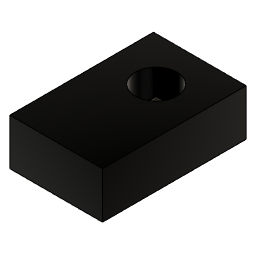
AMS_AS7341 (Autodesk Fusion 360 design; units mm, degrees)
Autodesk Fusion 360 part; units mm, degrees
note: some values were not read from the file. Set by a fixed rule: which face or edge a step refers to.
sketch "Sketch1" plane through (0, 0, 0) normal (0, 0, 1) x (1, 0, 0) in component "Body"
  line L0 (1, -1.55) -> (-1, -1.55)
  line L1 (-1, -1.55) -> (-1, 1.55)
  line L2 (-1, 1.55) -> (1, 1.55)
  line L3 (1, 1.55) -> (1, -1.55)
  line L4 (1, -1.55) -> (-1, 1.55) construction
  line L5 (-1, -1.55) -> (1, 1.55) construction
  dimension "d1" = 2
  dimension "d2" = 3.1
  constraint horizontal L0
  constraint perpendicular L0 L1
  constraint parallel L0 L2
  constraint parallel L1 L3
  constraint coincident L4 origin
  constraint coincident L5 origin
  measures "d1" distance of L1.end L2.end
  measures "d2" distance of L0.end L1.end
extrude "Extrude1" add sketch "Sketch1" along normal blind 1 makes body 1 in component "Body"
sketch "Sketch2" plane through (0, 0, 1) normal (0, 0, 1) x (-1, 0, 0) in component "Body"
  line L0 (-1, -1.55) -> (1, -1.55)
  line L1 (1, -1.55) -> (1, 1.55)
  line L2 (1, 1.55) -> (-1, 1.55)
  line L3 (-1, 1.55) -> (-1, -1.55)
  line L4 (0, 0) -> (0, -1.55) construction
  circle A0 centre (0, -0.609) radius 0.45
  dimension "d5" = 0.9
  dimension "d6" = 0.609
  constraint coincident L4.start origin
  constraint midpoint L0 L4.end
  constraint coincident L4 A0.centre
  measures "d5" diameter of A0
  measures "d6" distance of L4.start A0.centre
extrude "Extrude2" cut sketch "Sketch2" against normal blind 0.6 contours A0 bodies 1 in component "Body"
sketch "Sketch3" plane through (0, 0, 0) normal (0, 0, -1) x (1, 0, 0) in component "Body"
  line L0 (-1, -1.55) -> (1, -1.55)
  line L1 (1, -1.55) -> (1, 1.55)
  line L2 (1, 1.55) -> (-1, 1.55)
  line L3 (-1, 1.55) -> (-1, -1.55)
  line L4 (0, 1.55) -> (0, -1.55) construction
  line L5 (-1, 0) -> (1, 0) construction
  line L6 (-0.3505, 0.956) -> (-0.9255, 0.956)
  line L7 (-0.9255, 0.956) -> (-0.9255, 1.444)
  line L8 (-0.9255, 1.444) -> (-0.3505, 1.444)
  line L9 (-0.3505, 1.444) -> (-0.3505, 0.956)
  line L10 (-0.3505, 0.956) -> (-0.9255, 1.444) construction
  line L11 (-0.9255, 0.956) -> (-0.3505, 1.444) construction
  point P0 (-0.638, 1.2)
  dimension "d9" = 0.575
  dimension "d10" = 0.488
  dimension "d11" = 1.2
  dimension "d12" = 0.638
  dimension "d13" = 0.0745
  dimension "d14" = 0.106
  constraint midpoint L2 L4.start
  constraint midpoint L0 L4.end
  constraint midpoint L3 L5.start
  constraint midpoint L1 L5.end
  constraint horizontal L6
  constraint perpendicular L6 L7
  constraint parallel L6 L8
  constraint parallel L7 L9
  constraint coincident L10 P0
  constraint coincident L11 P0
  measures "d9" distance of L7.end L8.end
  measures "d10" distance of L6.end L7.end
  measures "d11" vertical distance of L5.start P0
  measures "d12" horizontal distance of L4.start P0
  measures "d13" horizontal distance of L2.end L7.end
  measures "d14" vertical distance of L2.end L7.end
extrude "Extrude3" cut sketch "Sketch3" against normal blind 0.05 contours L6 L7 L8 L9 bodies 1 in component "Body"
pattern_linear "R-Pattern1" count 2 spacing 1.276 along (1, 0, 0) count 4 spacing 0.8 along (0, 1, 0) of "Extrude3" in component "Body"
sketch "Sketch4" plane through (0, 0, 0.05) normal (0, 0, -1) x (1, 0, 0) in component "Body"
  line L0 (-0.3505, -0.956) -> (-0.9255, -0.956)
  line L1 (-0.9255, -0.956) -> (-0.9255, -1.444)
  line L2 (-0.9255, -1.444) -> (-0.3505, -1.444)
  line L3 (-0.3505, -1.444) -> (-0.3505, -0.956)
  line L4 (-0.3505, -1.1328) -> (-0.5273, -0.956)
  line L5 (-0.5273, -0.956) -> (-0.3505, -0.956)
  line L6 (-0.3505, -0.956) -> (-0.3505, -1.1328)
  dimension "d21" = 45
  dimension "d22" = 0.25
  constraint coincident L3 L4.start
  constraint coincident L0 L4.end
  constraint coincident L0.start L3.end
  constraint equal L5 L6
  measures "d21" angle of L4 L6
  measures "d22" distance of L4.start L4.end
extrude "Extrude4" add sketch "Sketch4" along normal up to surface (0.05 mm away) contours L0 L3 L4 L5 L6 bodies 1 in component "Body"
extrude "Extrude1'" add 8 faces at (0.5422, 1.1187, 0.05) (0.5422, 0.3187, 0.05) (0.5422, -0.4813, 0.05) (0.5422, -1.2813, 0.05) (-0.7338, -1.2813, 0.05) (-0.7338, -0.4813, 0.05) (-0.7338, 0.3187, 0.05) (-0.7928, 1.1187, 0.05) along direction (0, 0, -1) blind 0.06 separate body on bodies 1 makes body 2 at (-0.7338, 0.3187, 0.05) makes body 3 at (-0.7338, -1.2813, 0.05) makes body 4 at (0.5422, -0.4813, 0.05) makes body 5 at (0.5422, 1.1187, 0.05) makes body 6 at (0.5422, 0.3187, 0.05) makes body 7 at (0.5422, -1.2813, 0.05) makes body 8 at (-0.7338, -0.4813, 0.05) makes body 9 at (-0.7928, 1.1187, 0.05) in component "Pads"
sketch "Sketch1 (2)" plane through (0, 0, 0.4) normal (0, 0, 1) x (-1, 0, 0) in component "Photodiode"
  circle A0 centre (0, -0.609) radius 0.45
  circle A1 centre (0, -0.609) radius 0.45
  line L0 (-0.3182, -0.2908) -> (0.3182, -0.2908)
  line L1 (0.3182, -0.2908) -> (0.3182, -0.9272)
  line L2 (0.3182, -0.9272) -> (-0.3182, -0.9272)
  line L3 (-0.3182, -0.9272) -> (-0.3182, -0.2908)
  line L4 (-0.3182, -0.2908) -> (0.3182, -0.9272) construction
  line L5 (0.3182, -0.2908) -> (-0.3182, -0.9272) construction
  point P0 (0, -0.609)
  constraint horizontal L0
  constraint perpendicular L0 L1
  constraint parallel L0 L2
  constraint parallel L1 L3
  constraint coincident A1 L0.start
  constraint coincident L4 P0
  constraint coincident L5 P0
  constraint coincident P0 A0.centre
  constraint equal L2 L3
extrude "Extrude1''" add sketch "Sketch1 (2)" along normal blind 0.05 separate body contours L0 L1 L2 L3 makes body 10 in component "Photodiode"
component "Body" placed x (1, 0, 0) y (0, 1, 0) z (0, 0, 1) at (0, 0, 0)
component "Pads" placed x (1, 0, 0) y (0, 1, 0) z (0, 0, 1) at (0, 0, 0)
component "Photodiode" placed x (1, 0, 0) y (0, 1, 0) z (0, 0, 1) at (0, 0, 0)
